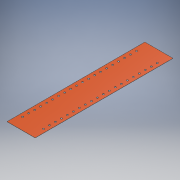
# Autodesk Inventor part: Skin NPS 6 Internal
Saved by Autodesk Inventor 2019 (Build 230136000, 136)
## iProperties
Created: 2016-08-30
Part Number: Skin NPS 6 Internal
Material: Rubber, Silicone
Document SubType Name: Modeling
Designer: IEUser
Density: 1.25 g/cm^3
Appearance: Rubber - Black
Author: IEUser
Autodesk Inventor part; units mm, degrees
ref_plane "YZ Plane" through (0, 0, 0) normal (1, 0, 0) x (0, 1, 0)
ref_plane "XZ Plane" through (0, 0, 0) normal (0, 1, 0) x (-1, 0, 0)
ref_plane "XY Plane" through (0, 0, 0) normal (0, 0, 1) x (1, 0, 0)
sketch "Skin Scheme" plane through (0, 0, 0) normal (0, 1, 0) x (-1, 0, 0)
  line L0 (464, -84.5) -> (-464, -84.5)
  line L1 (-464, -84.5) -> (-464, 84.5)
  line L2 (-464, 84.5) -> (464, 84.5)
  line L3 (464, 84.5) -> (464, -84.5)
  circle A0 centre (342, -62.5) radius 5
  circle A1 centre (306, -62.5) radius 5
  circle A2 centre (270, -62.5) radius 5
  circle A3 centre (234, -62.5) radius 5
  circle A4 centre (198, -62.5) radius 5
  circle A5 centre (162, -62.5) radius 5
  circle A6 centre (126, -62.5) radius 5
  circle A7 centre (90, -62.5) radius 5
  circle A8 centre (54, -62.5) radius 5
  circle A9 centre (18, -62.5) radius 5
  circle A10 centre (-18, -62.5) radius 5
  circle A11 centre (-54, -62.5) radius 5
  circle A12 centre (-90, -62.5) radius 5
  circle A13 centre (-126, -62.5) radius 5
  circle A14 centre (-162, -62.5) radius 5
  circle A15 centre (-198, -62.5) radius 5
  circle A16 centre (-234, -62.5) radius 5
  circle A17 centre (-270, -62.5) radius 5
  circle A18 centre (342, 62.5) radius 5
  circle A19 centre (306, 62.5) radius 5
  circle A20 centre (270, 62.5) radius 5
  circle A21 centre (234, 62.5) radius 5
  circle A22 centre (198, 62.5) radius 5
  circle A23 centre (162, 62.5) radius 5
  circle A24 centre (126, 62.5) radius 5
  circle A25 centre (90, 62.5) radius 5
  circle A26 centre (54, 62.5) radius 5
  circle A27 centre (18, 62.5) radius 5
  circle A28 centre (-18, 62.5) radius 5
  circle A29 centre (-54, 62.5) radius 5
  circle A30 centre (-90, 62.5) radius 5
  circle A31 centre (-126, 62.5) radius 5
  circle A32 centre (-162, 62.5) radius 5
  circle A33 centre (-198, 62.5) radius 5
  circle A34 centre (-234, 62.5) radius 5
  circle A35 centre (-270, 62.5) radius 5
  circle A36 centre (-306, -62.5) radius 5
  circle A37 centre (-306, 62.5) radius 5
  circle A38 centre (-342, -62.5) radius 5
  circle A39 centre (-342, 62.5) radius 5
  point P0 (0, 0)
  dimension "d0" = 928
  dimension "d1" = 464
  dimension "d2" = 169
  dimension "d3" = 84.5
  dimension "d4" = 10
  dimension "d5" = 122
  dimension "d6" = 22
  dimension "d9" = 36
  dimension "d12" = 125
  constraints: 40 centre point, 8 end point, 2 horizontal, 2 parallel, 1 perpendicular, 1 vertical, 78 other
  measures "d0" distance of L0.start L0.end
  measures "d1" distance from line of point (0, 0) L3
  measures "d2" distance of L2.end L0.start
  measures "d3" distance from line of point (0, 0) L0
  measures "d4" diameter of A0
  measures "d5" distance from line of L3 A0.centre
  measures "d6" distance from line of L0 A0.centre
  measures "d9" distance of A0.centre A1.centre
  measures "d12" distance of A0.centre A18.centre
extrude "Skin Body" add sketch "Skin Scheme" along normal blind 1
sketch "End Cut Outline" plane through (0, 1, 0) normal (0, 1, 0) x (1, 0, 0)
  line L0 (-414, 94.5) -> (-474, 94.5)
  line L1 (-474, 94.5) -> (-474, -94.5)
  line L2 (-474, -94.5) -> (-414, -94.5)
  line L3 (-414, -94.5) -> (-414, 94.5)
  line L4 (464, 84.5) -> (-464, 84.5) projected
  line L5 (-464, -84.5) -> (464, -84.5) projected
  line L6 (-464, 84.5) -> (-464, -84.5) projected
  point P0 (0, 0)
  dimension "d19" = 10
  dimension "d20" = 10
  dimension "d21" = 10
  dimension "d22" = 50
  constraints: 8 end point, 2 parallel, 1 horizontal, 1 perpendicular
  measures "d19" distance between parallel lines of L4 L0
  measures "d20" distance between parallel lines of L5 L2
  measures "d21" distance between parallel lines of L6 L1
  measures "d22" distance between parallel lines of L3 L6
extrude "End Cut" cut sketch "End Cut Outline" along normal through all both and the other way through all
mirror "End Cut Mirror" about plane through (0, 0, 0) normal (1, 0, 0) of "End Cut"
equation "\"d1\" = 0.5 * d0"
equation "\"d3\" = 0.5 * d2"
body "Solid2"
